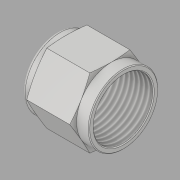
# Autodesk Inventor part: AN818-8D
Saved by Autodesk Inventor 2019 (Build 230136000, 136)
## iProperties
Created: 2018-11-23
Part Number: AN818-8D
Material: Aluminum 2014-T6
Document SubType Name: Modeling
Designer: erics
Density: 2.78927 g/cm^3
Appearance: Satin
Mass: 8.78984 g
Surface Area: 32.8467 cm^2
Volume: 3.1513 cm^3
Author: erics
Autodesk Inventor part; units mm, degrees
ref_plane "YZ Plane" through (0, 0, 0) normal (1, 0, 0) x (0, 1, 0)
ref_plane "XZ Plane" through (0, 0, 0) normal (0, 1, 0) x (-1, 0, 0)
ref_plane "XY Plane" through (0, 0, 0) normal (0, 0, 1) x (1, 0, 0)
sketch "Sketch1" plane through (0, 0, 0) normal (0, 0, 1) x (1, 0, 0)
  line L0 (1.1938, -11.1125) -> (21.3106, -11.1125)
  line L1 (21.5646, -10.8585) -> (21.5646, -9.779)
  line L2 (21.3106, -9.525) -> (3.4544, -9.525)
  line L3 (3.2004, -9.271) -> (3.2004, -7.493)
  line L4 (2.9464, -7.239) -> (0.254, -7.239)
  line L5 (0, -9.9187) -> (0, -7.493)
  arc A0 (0, -9.9187) -> (1.1938, -11.1125) centre (1.1938, -9.9187) ccw
  line L6 (0.254, -7.239) -> (0, -7.493)
  line L7 (2.9464, -7.239) -> (3.2004, -7.493)
  line L8 (21.3106, -11.1125) -> (21.5646, -10.8585)
  line L9 (21.3106, -9.525) -> (21.5646, -9.779)
  arc A1 (3.2004, -9.271) -> (3.4544, -9.525) centre (3.4544, -9.271) ccw
  line L10 (-4.6096, 0) -> (25.927, 0) projected
  point P0 (0, 0)
  point P1 (0, -11.1125)
  point P2 (21.5646, -11.1125)
  point P3 (21.5646, -9.525)
  point P4 (3.2004, -9.525)
  point P5 (3.2004, -7.239)
  point P6 (0, -7.239)
  dimension "d0" = 7.239
  dimension "d1" = 11.1125
  dimension "d2" = 21.5646
  dimension "d3" = 18.3642
  dimension "d4" = 1.1938
  dimension "d5" = 0.254
  dimension "d6" = 0.254
  dimension "d7" = 0.254
  dimension "d8" = 0.254
  dimension "d9" = 0.254
  dimension "d10" = 0.254
  dimension "d11" = 0.254
  dimension "d12" = 0.254
  dimension "d13" = 0.254
  dimension "d14" = 9.525
  constraints: 20 end point, 12 point on line, 4 perpendicular, 4 point on circle, 4 tangent, 2 centre point, 2 vertical alignment, 1 horizontal, 1 vertical
  measures "d0" distance from line of point (0, 0) L4
  measures "d1" distance from line of point (0, 0) L0
  measures "d2" distance of point (0, -11.113) point (21.565, -11.113)
  measures "d3" distance of point (21.565, -9.525) point (3.2, -9.525)
  measures "d4" radius of A0
  measures "d5" distance of L4.end point (0, -7.239)
  measures "d6" distance of L5.end point (0, -7.239)
  measures "d7" distance of L4.start point (3.2, -7.239)
  measures "d8" distance of L3.end point (3.2, -7.239)
  measures "d9" distance of L0.end point (21.565, -11.113)
  measures "d10" distance of L1.start point (21.565, -11.113)
  measures "d11" distance of L2.start point (21.565, -9.525)
  measures "d12" distance of L1.end point (21.565, -9.525)
  measures "d13" radius of A1
  measures "d14" distance from line of point (0, 0) L2
revolve "Revolution1" add sketch "Sketch1" angle 360 about axis through (-10, 0, 0) along (1, 0, 0)
ref_plane "Work Plane1" through (17.6022, 0, 0) normal (1, 0, 0) x (0, 0, -1)
sketch "Sketch2" plane through (17.6022, 0, 0) normal (1, 0, 0) x (0, 0, -1)
  circle A0 centre (0, 0) radius 9.525 projected
  circle A1 centre (0, 0) radius 11.1125 projected
  line L0 (6.4158, 11.1125) -> (12.8316, 0)
  line L1 (12.8316, 0) -> (6.4158, -11.1125)
  line L2 (6.4158, -11.1125) -> (-6.4158, -11.1125)
  line L3 (-6.4158, -11.1125) -> (-12.8316, 0)
  line L4 (-12.8316, 0) -> (-6.4158, 11.1125)
  line L5 (-6.4158, 11.1125) -> (6.4158, 11.1125)
  dimension "d24" = 22.225
  constraints: 12 end point, 1 coincident, 1 horizontal, 13 other
  measures "d24" distance between parallel lines of L2 L5
extrude "Extrusion1" add sketch "Sketch2" against normal blind 14.6812 contours A1 L0 L1 | A1 L5 L0 | L1 L2 A1 | A1 L4 L5 | L2 L3 A1 | A1 L3 L4
sketch "Sketch3" plane through (0, 0, 0) normal (0, 1, 0) x (-1, 0, 0)
  line L0 (-21.3106, 11.1125) -> (-17.6022, 11.1125) construction
  line L1 (-17.6022, 6.4158) -> (-17.6022, 12.8316) construction
  line L2 (-2.921, 6.4158) -> (-2.921, 9.6237) construction
  line L3 (-17.6022, 6.4158) -> (-2.921, 6.4158) construction
  line L4 (-17.6022, 6.4158) -> (-17.6022, 9.6237) construction
  line L5 (-17.6022, 12.8316) -> (-2.921, 12.8316) construction
  line L6 (-2.921, 11.1125) -> (-1.1938, 11.1125) construction
  line L7 (-17.6022, 11.1125) -> (-17.1416, 12.8316)
  line L8 (-2.921, 11.1125) -> (-3.3816, 12.8316)
  line L9 (4.2621, 0) -> (-25.5727, 0) projected
  line L10 (-2.921, 11.1125) -> (-2.921, 12.8316)
  line L11 (-3.3816, 12.8316) -> (-2.921, 12.8316)
  line L12 (-17.1416, 12.8316) -> (-17.6022, 12.8316)
  line L13 (-17.6022, 11.1125) -> (-17.6022, 12.8316)
  line L14 (-17.6022, 9.6237) -> (-17.6022, 12.8316) projected
  line L15 (-2.921, 9.6237) -> (-2.921, 12.8316) projected
  point P0 (0, 0)
  dimension "d19" = 15
  dimension "d25" = 15
  constraints: 12 end point, 2 collinear, 2 point on line, 1 perpendicular, 1 vertical
  measures "d19" angle of L1 L7
  measures "d25" angle of L2 L8
revolve "Revolution2" cut sketch "Sketch3" angle 360 about axis through (-10, 0, 0) along (1, 0, 0)
thread "Thread1" size "3/4-16 UNF" class "3B" standard "ANSI Unified Screw Threads" length 16.4338
equation "\"d0\" = 0.5 * AN818_A"
equation "\"d1\" = 0.5 * AN818_C"
equation "\"d2\" = AN818_M"
equation "\"d3\" = AN818_L"
equation "\"d4\" = AN818_R"
equation "\"d5\" = AN818_U"
equation "\"d6\" = d5"
equation "\"d7\" = d5"
equation "\"d8\" = d7"
equation "\"d9\" = AN818_N"
equation "\"d10\" = d9"
equation "\"d11\" = d9"
equation "\"d12\" = d11"
equation "\"d14\" = 0.5 * Thread"
equation "\"d24\" = AN818_P"
equation "\"d17\" = AN818_J"
equation "\"d22\" = AN818_S"
equation "\"AN818_A\" = 14.478"
equation "\"AN818_B\" = 3.9624"
equation "\"AN818_C\" = 22.225"
equation "\"AN818_H\" = 19.05"
equation "\"AN818_J\" = 14.6812"
equation "\"AN818_L\" = 18.3642"
equation "\"AN818_M\" = 21.5646"
equation "\"AN818_N\" = 0.254"
equation "\"AN818_P\" = 22.225"
equation "\"AN818_Q\" = 12.2936"
equation "\"AN818_R\" = 1.1938"
equation "\"AN818_S\" = 16.4338"
equation "\"AN818_U\" = 0.254"
equation "\"Thread\" = 19.05"
equation "\"d16\" = -AN818_B"
equation "\"Tube_OD\" = 12.7"
body "Solid1"
